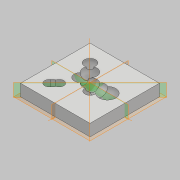
# Autodesk Inventor part: Placa - Daños Esfera
Saved by Autodesk Inventor 2017 (Build 210142000, 142)
## iProperties
Part Number: Placa - Daños Esfera
Material: Genérico
Document SubType Name: Modeling
Designer: franc
Density: 1 g/cm^3
Appearance: Valor por defecto
Author: franc
Autodesk Inventor part; units mm, degrees
sketch "Boceto1" plane through (0, 0, 0) normal (0, 0, 1) x (1, 0, 0)
  line L0 (-75, 75) -> (75, 75)
  line L1 (75, 75) -> (75, -75)
  line L2 (75, -75) -> (-75, -75)
  line L3 (-75, -75) -> (-75, 75)
  line L4 (-75, 75) -> (75, -75) construction
  line L5 (75, 75) -> (-75, -75) construction
  point P0 (0, 0)
  dimension "d0" = 150
  dimension "d1" = 150
  constraints: 12 end point, 2 midpoint, 2 parallel, 1 horizontal, 1 perpendicular
  measures "d0" distance of L1.end L2.end
  measures "d1" distance of L0.end L1.end
extrude "Extrusión1" add sketch "Boceto1" along normal blind 25.4
sketch "Boceto3" plane through (0, 0, 0) normal (0, 1, 0) x (-1, 0, 0)
  line L0 (-75, 25.4) -> (75, 25.4) projected
  arc A0 (-15, 25.4) -> (15, 25.4) centre (0, 25.4) ccw
  line L1 (15, 25.4) -> (-15, 25.4)
  point P0 (0, 0)
  dimension "d7" = 15
  constraints: 2 end point, 2 point on circle, 1 centre point, 1 collinear, 1 midpoint, 1 point on line
  measures "d7" radius of A0
revolve "Revolución2" cut sketch "Boceto3" angle 360 about axis through (75, 0, 25.4) along (-1, 0, 0)
ref_plane "Plano de trabajo1" through (-75, -75, 0) normal (-0.7071, 0.7071, 0) x (0, 0, 1)
ref_plane "Plano de trabajo2" through (75, -75, 0) normal (-0.7071, -0.7071, 0) x (0, 0, 1)
sketch "Boceto4" plane through (-75, -75, 0) normal (-0.7071, 0.7071, 0) x (0, 0, 1)
  line L0 (25.4, 106.066) -> (25.4, 0) projected
  arc A0 (25.4, 68.9087) -> (25.4, 48.9087) centre (25.4, 58.9087) ccw
  line L1 (25.4, 48.9087) -> (25.4, 68.9087)
  point P0 (0, 106.066)
  dimension "d11" = 10
  constraints: 2 end point, 2 point on circle, 2 point on line, 1 centre point, 1 collinear
  measures "d11" radius of A0
sketch "Boceto5" plane through (75, -75, 0) normal (-0.7071, -0.7071, 0) x (0, 0, 1)
  line L0 (25.4, 106.066) -> (25.4, 212.132) projected
  arc A0 (25.4, 171.8235) -> (25.4, 147.8235) centre (25.4, 159.8235) ccw
  line L1 (25.4, 171.8235) -> (25.4, 147.8235)
  point P0 (0, 106.066)
  dimension "d12" = 12
  constraints: 2 end point, 2 point on circle, 2 point on line, 1 centre point, 1 vertical
  measures "d12" radius of A0
sketch "Boceto6" plane through (0, 0, 0) normal (0, 1, 0) x (-1, 0, 0)
  arc A0 (-55.646, 25.4) -> (-19.646, 25.4) centre (-37.646, 25.4) ccw
  line L0 (-19.646, 25.4) -> (-55.646, 25.4)
  line L1 (-75, 25.4) -> (75, 25.4) projected
  point P0 (0, 0)
  dimension "d13" = 18
  constraints: 2 end point, 2 point on circle, 1 centre point, 1 collinear
  measures "d13" radius of A0
revolve "Revolución3" cut sketch "Boceto5" angle 360 about axis through (0, 0, 25.4) along (-0.7071, 0.7071, 0)
revolve "Revolución4" cut sketch "Boceto4" angle 360 about axis through (0, 0, 25.4) along (-0.7071, -0.7071, 0)
revolve "Revolución5" cut sketch "Boceto6" angle 360 about axis through (19.646, 0, 25.4) along (1, 0, 0)
sketch "Boceto7" plane through (0, 0, 0) normal (0, 1, 0) x (-1, 0, 0)
  line L0 (-75, 25.4) -> (75, 25.4) projected
  arc A0 (-33.0988, 25.4) -> (-3.0988, 25.4) centre (-18.0988, 25.4) ccw
  line L1 (-3.0988, 25.4) -> (-33.0988, 25.4)
  line L2 (-55.646, 25.4) -> (-19.646, 25.4) projected
  point P0 (0, 0)
  dimension "d17" = 15
  constraints: 2 end point, 2 point on circle, 2 point on line, 1 centre point, 1 collinear
  measures "d17" radius of A0
revolve "Revolución6" cut sketch "Boceto7" angle 360 about axis through (3.0988, 0, 25.4) along (1, 0, 0)
sketch "Boceto9" plane through (75, -75, 0) normal (-0.7071, -0.7071, 0) x (0, 0, 1)
  line L0 (25.4, 106.066) -> (25.4, 0) projected
  arc A0 (25.4, 96.0806) -> (25.4, 74.0806) centre (25.4, 85.0806) ccw
  line L1 (25.4, 96.0806) -> (25.4, 74.0806)
  point P0 (0, 106.066)
  dimension "d19" = 11
  constraints: 2 end point, 2 point on circle, 2 point on line, 1 centre point, 1 collinear
  measures "d19" radius of A0
revolve "Revolución7" cut sketch "Boceto9" angle 360 about axis through (0, 0, 25.4) along (0.7071, -0.7071, 0)
sketch "Boceto10" plane through (-75, -75, 0) normal (-0.7071, 0.7071, 0) x (0, 0, 1)
  line L0 (25.4, 106.066) -> (25.4, 0) projected
  arc A0 (25.4, 58.9481) -> (25.4, 38.9481) centre (25.4, 48.9481) ccw
  line L1 (25.4, 38.9481) -> (25.4, 58.9481)
  line L2 (25.4, 68.9087) -> (25.4, 48.9087) projected
  arc A1 (25.4, 54.0246) -> (25.4, 34.0246) centre (25.4, 44.0246) ccw
  line L3 (25.4, 34.0246) -> (25.4, 54.0246)
  point P0 (0, 106.066)
  dimension "d21" = 10
  dimension "d22" = 10
  constraints: 4 end point, 4 point on circle, 4 point on line, 2 centre point, 1 collinear, 1 vertical
  measures "d21" radius of A0
  measures "d22" radius of A1
revolve "Revolución8" cut sketch "Boceto10" angle 360 about axis through (0, 0, 25.4) along (-0.7071, -0.7071, 0)
sketch "Boceto11" plane through (75, -75, 0) normal (-0.7071, -0.7071, 0) x (0, 0, 1)
  line L0 (25.4, 212.132) -> (25.4, 106.066) projected
  arc A0 (25.4, 150.634) -> (25.4, 120.634) centre (25.4, 135.634) ccw
  line L1 (25.4, 120.634) -> (25.4, 150.634)
  point P0 (0, 106.066)
  dimension "d24" = 15
  constraints: 2 end point, 2 point on circle, 2 point on line, 1 centre point, 1 vertical
  measures "d24" radius of A0
revolve "Revolución9" cut sketch "Boceto11" angle 360 about axis through (-75, 75, 25.4) along (0.7071, -0.7071, 0)
sketch "Boceto12" plane through (0, 0, 0) normal (0, 1, 0) x (-1, 0, 0)
  line L0 (23.3453, 25.4) -> (42.9986, 25.4) projected
  arc A0 (8.2719, 25.4) -> (34.2719, 25.4) centre (21.2719, 25.4) ccw
  line L1 (8.2719, 25.4) -> (34.2719, 25.4)
  line L2 (75, 25.4) -> (-75, 25.4) projected
  point P0 (0, 0)
  point P1 (30.7351, 25.4)
  dimension "d26" = 13
  constraints: 2 end point, 2 point on circle, 1 centre point, 1 collinear, 1 point on line
  measures "d26" radius of A0
revolve "Revolución10" cut sketch "Boceto12" angle 360 about axis through (-23.3453, 0, 25.4) along (-1, 0, 0)
